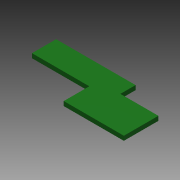
# Autodesk Inventor part: MezzanineBoard
Saved by Autodesk Inventor 2014 (Build 180170000, 170)
## iProperties
Created: 2015-11-05
Part Number: MezzanineBoard
Material: Generic
Document SubType Name: Modeling
Designer: Owner
Density: 1 g/cm^3
Appearance: Smooth - Dark Forest Green
Author: Owner
Autodesk Inventor part; units mm, degrees
ref_plane "YZ Plane" through (0, 0, 0) normal (1, 0, 0) x (0, 1, 0)
ref_plane "XZ Plane" through (0, 0, 0) normal (0, 1, 0) x (-1, 0, 0)
ref_plane "XY Plane" through (0, 0, 0) normal (0, 0, 1) x (1, 0, 0)
sketch "Sketch1" plane through (0, 0, 0) normal (0, 1, 0) x (-1, 0, 0)
  line L0 (-14.7409, 9.4688) -> (28.4391, 9.4688)
  line L1 (28.4391, 9.4688) -> (28.4391, -8.8192)
  line L2 (28.4391, -8.8192) -> (-14.7409, -8.8192)
  line L3 (-14.7409, -8.8192) -> (-14.7409, 9.4688)
  line L4 (-14.7409, 9.4688) -> (7.3571, 9.4688)
  line L5 (7.3571, 9.4688) -> (7.3571, 0.0708)
  line L6 (-0.7709, -3.2312) -> (-14.7409, -3.2312)
  line L7 (-14.7409, -3.2312) -> (-14.7409, 9.4688)
  line L8 (28.4391, -8.8192) -> (-0.7709, -8.8192)
  line L9 (-0.7709, -8.8192) -> (-0.7709, -3.2312)
  line L10 (7.3571, 0.0708) -> (28.4391, 0.0708)
  line L11 (28.4391, 0.0708) -> (28.4391, -8.8192)
  point P0 (0, 0)
  dimension "d0" = 43.18
  dimension "d1" = 18.288
  dimension "d2" = 13.97
  dimension "d3" = 21.082
  dimension "d4" = 5.588
  dimension "d5" = 9.398
  constraints: 24 end point, 6 parallel, 3 horizontal, 3 perpendicular
  measures "d0" distance of L0.start L0.end
  measures "d1" distance of L2.end L0.start
  measures "d2" distance of L6.start L6.end
  measures "d3" distance of L5.end L10.end
  measures "d4" distance of L8.end L6.start
  measures "d5" distance of L4.end L5.end
extrude "Extrusion1" add sketch "Sketch1" along normal blind 1.6 contours L0 L5 L10 L1 L2 L9 L6 L3
body "Solid1"
